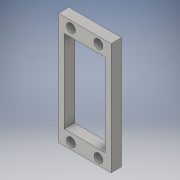
# Autodesk Inventor part: JBTable2Draft
Saved by Autodesk Inventor 2016 (Build 200138000, 138)
## iProperties
Created: 2017-05-18
Part Number: JBTable2Draft
Material: Generic
Document SubType Name: Modeling
Designer: Student
Density: 1 g/cm^3
Appearance: Default
Author: Student
Autodesk Inventor part; units mm, degrees
ref_plane "YZ Plane" through (0, 0, 0) normal (1, 0, 0) x (0, 1, 0)
ref_plane "XZ Plane" through (0, 0, 0) normal (0, 1, 0) x (-1, 0, 0)
ref_plane "XY Plane" through (0, 0, 0) normal (0, 0, 1) x (1, 0, 0)
sketch "Sketch1" plane through (0, 0, 0) normal (0, 0, 1) x (1, 0, 0)
  line L0 (-12.7, -26.924) -> (12.7, -26.924)
  line L1 (12.7, -26.924) -> (12.7, 26.924)
  line L2 (12.7, 26.924) -> (-12.7, 26.924)
  line L3 (-12.7, 26.924) -> (-12.7, -26.924)
  line L4 (-9.906, -19.939) -> (9.906, -19.939)
  line L5 (9.906, -19.939) -> (9.906, 19.939)
  line L6 (9.906, 19.939) -> (-9.906, 19.939)
  line L7 (-9.906, 19.939) -> (-9.906, -19.939)
  circle A0 centre (-6.6179, 23.7806) radius 2.155
  circle A1 centre (6.6179, 23.7806) radius 2.155
  circle A2 centre (-6.6179, -23.809) radius 2.155
  circle A3 centre (6.6179, -23.809) radius 2.155
  dimension "d0" = 25.4
  dimension "d1" = 53.848
  dimension "d3" = 39.878
  constraints: 16 end point, 4 centre point, 4 parallel, 2 horizontal, 2 perpendicular
  measures "d0" distance of L2.end L1.end
  measures "d1" distance of L1.end L0.end
  measures "d3" distance of L5.end L4.end
extrude "Extrusion1" add sketch "Sketch1" along normal blind 5.08
body "Solid1"
